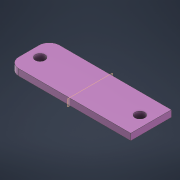
# Autodesk Inventor part: SideSensorCircuit
Saved by Autodesk Inventor 2022 (Build 260153000, 153)
## iProperties
Created: 2021-10-25
Part Number: SideSensorCircuit
Material: 一般
Document SubType Name: Modeling
Designer: shiok
Density: 1 g/cm^3
Appearance: 既定
Author: shiok
Autodesk Inventor part; units mm, degrees
ref_plane "XZ Plane" through (0, 0, 0) normal (0, 1, 0) x (-1, 0, 0)
ref_plane "XY Plane" through (0, 0, 0) normal (0, 0, 1) x (1, 0, 0)
sketch "スケッチ1" plane through (0, 0, 0) normal (0, 1, 0) x (-1, 0, 0)
  line L0 (15, -5) -> (-15, -5)
  line L1 (-15, -5) -> (-15, 5)
  line L2 (-15, 5) -> (15, 5)
  line L3 (15, 5) -> (15, -5)
  line L4 (-15, 5) -> (15, -5) construction
  line L5 (15, 5) -> (-15, -5) construction
  point P0 (0, 0)
  point P1 (0, 0)
  dimension "d1" = 10
  dimension "d13" = 15
  constraints: 12 end point, 2 midpoint, 2 parallel, 1 coincident, 1 horizontal, 1 perpendicular
  measures "d1" distance of L0.end L1.end
  measures "d13" distance from line of L3 point (0, 0)
extrude "押し出し1" add sketch "スケッチ1" along normal blind 1.6
sketch "スケッチ2" plane through (0, 1.6, 0) normal (0, 1, 0) x (1, 0, 0)
  line L0 (0, 0) -> (-12.25, 0) construction
  line L1 (15, 5) -> (-15, 5) projected
  line L2 (0, 5) -> (0, -5)
  line L3 (-15, -5) -> (15, -5) projected
  point P0 (12.25, 0)
  dimension "d4" = 12.25
  constraints: 4 end point, 2 midpoint, 1 coincident, 1 horizontal, 1 symmetric about line
  measures "d4" distance of L0.start L0.end
hole "穴1" at (-12.25, 1.6, 0) at (12.25, 1.6, 0) direction (0, -1, 0) diameter 2.4 depth 1.6 tip angle 118 clearance for "Countersunk Flat Head Screw ISO 2009/7046" size "M2" standard "ISO"
fillet "フィレット2" radius 2.5 2 edges at (-15, 0.8, 5) (-15, 0.8, -5)
